Autodesk Fusion 360 part; units mm, degrees
(part 3 of 3)
  line L1894 (31.4632, 18.5996) -> (31.4764, 18.5928)
  line L1895 (31.4764, 18.5928) -> (31.4891, 18.5858)
  line L1896 (31.4891, 18.5858) -> (31.5018, 18.5786)
  line L1897 (31.5018, 18.5786) -> (31.5145, 18.5712)
  line L1898 (31.5145, 18.5712) -> (31.527, 18.5635)
  line L1899 (31.527, 18.5635) -> (31.5394, 18.5556)
  line L1900 (31.5394, 18.5556) -> (31.5516, 18.5475)
  line L1901 (31.5516, 18.5475) -> (31.5637, 18.5392)
  line L1902 (31.5637, 18.5392) -> (31.5756, 18.5307)
  line L1903 (31.5756, 18.5307) -> (31.5875, 18.522)
  line L1904 (31.5875, 18.522) -> (31.5992, 18.5131)
  line L1905 (31.5992, 18.5131) -> (31.6106, 18.504)
  line L1906 (31.6106, 18.504) -> (31.6219, 18.4946)
  line L1907 (31.6219, 18.4946) -> (31.6331, 18.4851)
  line L1908 (31.6331, 18.4851) -> (31.6439, 18.4754)
  line L1909 (31.6439, 18.4754) -> (31.6547, 18.4655)
  line L1910 (31.6547, 18.4655) -> (31.6656, 18.4554)
  line L1911 (31.6656, 18.4554) -> (31.6759, 18.4451)
  line L1912 (31.6759, 18.4451) -> (31.6862, 18.4347)
  line L1913 (31.6862, 18.4347) -> (31.6963, 18.424)
  line L1914 (31.6963, 18.424) -> (31.7061, 18.4132)
  line L1915 (31.7061, 18.4132) -> (31.7159, 18.4022)
  line L1916 (31.7159, 18.4022) -> (31.7254, 18.3911)
  line L1917 (31.7254, 18.3911) -> (31.7347, 18.3798)
  line L1918 (31.7347, 18.3798) -> (31.7439, 18.3683)
  line L1919 (31.7439, 18.3683) -> (31.7529, 18.3567)
  line L1920 (31.7529, 18.3567) -> (31.7616, 18.3449)
  line L1921 (31.7616, 18.3449) -> (31.7701, 18.3329)
  line L1922 (31.7701, 18.3329) -> (31.7783, 18.3209)
  line L1923 (31.7783, 18.3209) -> (31.7865, 18.3086)
  line L1924 (31.7865, 18.3086) -> (31.7944, 18.2963)
  line L1925 (31.7944, 18.2963) -> (31.8021, 18.2838)
  line L1926 (31.8021, 18.2838) -> (31.8095, 18.2711)
  line L1927 (31.8095, 18.2711) -> (31.8167, 18.2584)
  line L1928 (31.8167, 18.2584) -> (31.8236, 18.2455)
  line L1929 (31.8236, 18.2455) -> (31.8304, 18.2325)
  line L1930 (31.8304, 18.2325) -> (31.837, 18.2194)
  line L1931 (31.837, 18.2194) -> (31.8434, 18.2061)
  line L1932 (31.8434, 18.2061) -> (31.8495, 18.1928)
  line L1933 (31.8495, 18.1928) -> (31.8553, 18.1793)
  line L1934 (31.8553, 18.1793) -> (31.8609, 18.1658)
  line L1935 (31.8609, 18.1658) -> (31.8662, 18.1522)
  line L1936 (31.8662, 18.1522) -> (31.8714, 18.1384)
  line L1937 (31.8714, 18.1384) -> (31.8762, 18.1246)
  line L1938 (31.8762, 18.1246) -> (31.881, 18.1107)
  line L1939 (31.881, 18.1107) -> (31.8852, 18.0967)
  line L1940 (31.8852, 18.0967) -> (31.8894, 18.0827)
  line L1941 (31.8894, 18.0827) -> (31.8934, 18.0685)
  line L1942 (31.8934, 18.0685) -> (31.8971, 18.0543)
  line L1943 (31.8971, 18.0543) -> (31.9005, 18.0401)
  line L1944 (31.9005, 18.0401) -> (31.9037, 18.0258)
  line L1945 (31.9037, 18.0258) -> (31.9066, 18.0114)
  line L1946 (31.9066, 18.0114) -> (31.9093, 17.997)
  line L1947 (31.9093, 17.997) -> (31.9117, 17.9825)
  line L1948 (31.9117, 17.9825) -> (31.9138, 17.968)
  line L1949 (31.9138, 17.968) -> (31.9156, 17.9535)
  line L1950 (31.9156, 17.9535) -> (31.9175, 17.9389)
  line L1951 (31.9175, 17.9389) -> (31.9188, 17.9243)
  line L1952 (31.9188, 17.9243) -> (31.9199, 17.9097)
  line L1953 (31.9199, 17.9097) -> (31.9209, 17.8951)
  line L1954 (31.9209, 17.8951) -> (31.9215, 17.8804)
  line L1955 (31.9215, 17.8804) -> (31.922, 17.8658)
  line L1956 (31.922, 17.8658) -> (31.922, 17.8511)
  line L1957 (31.922, 17.8511) -> (31.922, 6.9304)
  line L1958 (31.922, 6.9304) -> (31.922, 6.9158)
  line L1959 (31.922, 6.9158) -> (31.9215, 6.9011)
  line L1960 (31.9215, 6.9011) -> (31.9209, 6.8865)
  line L1961 (31.9209, 6.8865) -> (31.9199, 6.8718)
  line L1962 (31.9199, 6.8718) -> (31.9188, 6.8572)
  line L1963 (31.9188, 6.8572) -> (31.9175, 6.8426)
  line L1964 (31.9175, 6.8426) -> (31.9156, 6.828)
  line L1965 (31.9156, 6.828) -> (31.9138, 6.8135)
  line L1966 (31.9138, 6.8135) -> (31.9117, 6.799)
  line L1967 (31.9117, 6.799) -> (31.9093, 6.7846)
  line L1968 (31.9093, 6.7846) -> (31.9066, 6.7701)
  line L1969 (31.9066, 6.7701) -> (31.9037, 6.7558)
  line L1970 (31.9037, 6.7558) -> (31.9005, 6.7415)
  line L1971 (31.9005, 6.7415) -> (31.8971, 6.7272)
  line L1972 (31.8971, 6.7272) -> (31.8934, 6.713)
  line L1973 (31.8934, 6.713) -> (31.8894, 6.6989)
  line L1974 (31.8894, 6.6989) -> (31.8852, 6.6848)
  line L1975 (31.8852, 6.6848) -> (31.881, 6.6708)
  line L1976 (31.881, 6.6708) -> (31.8762, 6.6569)
  line L1977 (31.8762, 6.6569) -> (31.8714, 6.6431)
  line L1978 (31.8714, 6.6431) -> (31.8662, 6.6294)
  line L1979 (31.8662, 6.6294) -> (31.8609, 6.6157)
  line L1980 (31.8609, 6.6157) -> (31.8553, 6.6022)
  line L1981 (31.8553, 6.6022) -> (31.8495, 6.5888)
  line L1982 (31.8495, 6.5888) -> (31.8434, 6.5754)
  line L1983 (31.8434, 6.5754) -> (31.837, 6.5622)
  line L1984 (31.837, 6.5622) -> (31.8304, 6.549)
  line L1985 (31.8304, 6.549) -> (31.8236, 6.5361)
  line L1986 (31.8236, 6.5361) -> (31.8167, 6.5232)
  line L1987 (31.8167, 6.5232) -> (31.8095, 6.5104)
  line L1988 (31.8095, 6.5104) -> (31.8021, 6.4978)
  line L1989 (31.8021, 6.4978) -> (31.7944, 6.4853)
  line L1990 (31.7944, 6.4853) -> (31.7865, 6.4729)
  line L1991 (31.7865, 6.4729) -> (31.7783, 6.4607)
  line L1992 (31.7783, 6.4607) -> (31.7701, 6.4486)
  line L1993 (31.7701, 6.4486) -> (31.7616, 6.4367)
  line L1994 (31.7616, 6.4367) -> (31.7529, 6.4249)
  line L1995 (31.7529, 6.4249) -> (31.7439, 6.4132)
  line L1996 (31.7439, 6.4132) -> (31.7347, 6.4018)
  line L1997 (31.7347, 6.4018) -> (31.7254, 6.3905)
  line L1998 (31.7254, 6.3905) -> (31.7159, 6.3793)
  line L1999 (31.7159, 6.3793) -> (31.7061, 6.3683)
  line L2000 (31.7061, 6.3683) -> (31.6963, 6.3575)
  line L2001 (31.6963, 6.3575) -> (31.6862, 6.3469)
  line L2002 (31.6862, 6.3469) -> (31.6759, 6.3364)
  line L2003 (31.6759, 6.3364) -> (31.6656, 6.3261)
  line L2004 (31.6656, 6.3261) -> (31.6547, 6.3161)
  line L2005 (31.6547, 6.3161) -> (31.6439, 6.3062)
  line L2006 (31.6439, 6.3062) -> (31.6331, 6.2964)
  line L2007 (31.6331, 6.2964) -> (31.6219, 6.2869)
  line L2008 (31.6219, 6.2869) -> (31.6106, 6.2776)
  line L2009 (31.6106, 6.2776) -> (31.5992, 6.2685)
  line L2010 (31.5992, 6.2685) -> (31.5875, 6.2595)
  line L2011 (31.5875, 6.2595) -> (31.5756, 6.2508)
  line L2012 (31.5756, 6.2508) -> (31.5637, 6.2423)
  line L2013 (31.5637, 6.2423) -> (31.5516, 6.234)
  line L2014 (31.5516, 6.234) -> (31.5394, 6.2259)
  line L2015 (31.5394, 6.2259) -> (31.527, 6.218)
  line L2016 (31.527, 6.218) -> (31.5145, 6.2104)
  line L2017 (31.5145, 6.2104) -> (31.5018, 6.2029)
  line L2018 (31.5018, 6.2029) -> (31.4891, 6.1957)
  line L2019 (31.4891, 6.1957) -> (31.4764, 6.1887)
  line L2020 (31.4764, 6.1887) -> (31.4632, 6.1819)
  line L2021 (31.4632, 6.1819) -> (31.4502, 6.1754)
  line L2022 (31.4502, 6.1754) -> (31.437, 6.1691)
  line L2023 (31.437, 6.1691) -> (31.4235, 6.163)
  line L2024 (31.4235, 6.163) -> (31.4103, 6.1571)
  line L2025 (31.4103, 6.1571) -> (31.3965, 6.1515)
  line L2026 (31.3965, 6.1515) -> (31.383, 6.1462)
  line L2027 (31.383, 6.1462) -> (31.3693, 6.141)
  line L2028 (31.3693, 6.141) -> (31.3555, 6.1361)
  line L2029 (31.3555, 6.1361) -> (31.3415, 6.1315)
  line L2030 (31.3415, 6.1315) -> (31.3275, 6.1271)
  line L2031 (31.3275, 6.1271) -> (31.3134, 6.1229)
  line L2032 (31.3134, 6.1229) -> (31.2994, 6.119)
  line L2033 (31.2994, 6.119) -> (31.2851, 6.1153)
  line L2034 (31.2851, 6.1153) -> (31.2708, 6.1119)
  line L2035 (31.2708, 6.1119) -> (31.2566, 6.1087)
  line L2036 (31.2566, 6.1087) -> (31.2423, 6.1058)
  line L2037 (31.2423, 6.1058) -> (31.2277, 6.1031)
  line L2038 (31.2277, 6.1031) -> (31.2134, 6.1007)
  line L2039 (31.2134, 6.1007) -> (31.1989, 6.0985)
  line L2040 (31.1989, 6.0985) -> (31.1843, 6.0966)
  line L2041 (31.1843, 6.0966) -> (31.1698, 6.095)
  line L2042 (31.1698, 6.095) -> (31.1552, 6.0936)
  line L2043 (31.1552, 6.0936) -> (31.1404, 6.0924)
  line L2044 (31.1404, 6.0924) -> (31.1258, 6.0915)
  line L2045 (31.1258, 6.0915) -> (31.1113, 6.0909)
  line L2046 (31.1113, 6.0909) -> (31.0965, 6.0905)
  line L2047 (31.0965, 6.0905) -> (31.0819, 6.0904)
  line L2048 (31.0819, 6.0904) -> (3.7802, 6.0904)
  line L2049 (-0.0202, -1.1549) -> (-0.0403, -1.1544)
  line L2050 (-0.0403, -1.1544) -> (-0.0604, -1.1535)
  line L2051 (-0.0604, -1.1535) -> (-0.0806, -1.1523)
  line L2052 (-0.0806, -1.1523) -> (-0.1007, -1.1507)
  line L2053 (-0.1007, -1.1507) -> (-0.1207, -1.1487)
  line L2054 (-0.1207, -1.1487) -> (-0.1408, -1.1465)
  line L2055 (-0.1408, -1.1465) -> (-0.1608, -1.1438)
  line L2056 (-0.1608, -1.1438) -> (-0.1807, -1.1408)
  line L2057 (-0.1807, -1.1408) -> (-0.2006, -1.1375)
  line L2058 (-0.2006, -1.1375) -> (-0.2204, -1.1339)
  line L2059 (-0.2204, -1.1339) -> (-0.2402, -1.1298)
  line L2060 (-0.2402, -1.1298) -> (-0.2598, -1.1255)
  line L2061 (-0.2598, -1.1255) -> (-0.2794, -1.1208)
  line L2062 (-0.2794, -1.1208) -> (-0.299, -1.1157)
  line L2063 (-0.299, -1.1157) -> (-0.3184, -1.1103)
  line L2064 (-0.3184, -1.1103) -> (-0.3377, -1.1046)
  line L2065 (-0.3377, -1.1046) -> (-0.3569, -1.0985)
  line L2066 (-0.3569, -1.0985) -> (-0.3761, -1.0921)
  line L2067 (-0.3761, -1.0921) -> (-0.3951, -1.0854)
  line L2068 (-0.3951, -1.0854) -> (-0.4139, -1.0783)
  line L2069 (-0.4139, -1.0783) -> (-0.4327, -1.071)
  line L2070 (-0.4327, -1.071) -> (-0.4513, -1.0632)
  line L2071 (-0.4513, -1.0632) -> (-0.4698, -1.0552)
  line L2072 (-0.4698, -1.0552) -> (-0.4882, -1.0468)
  line L2073 (-0.4882, -1.0468) -> (-0.5063, -1.0382)
  line L2074 (-0.5063, -1.0382) -> (-0.5244, -1.0292)
  line L2075 (-0.5244, -1.0292) -> (-0.5423, -1.0199)
  line L2076 (-0.5423, -1.0199) -> (-0.56, -1.0102)
  line L2077 (-0.56, -1.0102) -> (-0.5775, -1.0003)
  line L2078 (-0.5775, -1.0003) -> (-0.5949, -0.9901)
  line L2079 (-0.5949, -0.9901) -> (-0.6121, -0.9796)
  line L2080 (-0.6121, -0.9796) -> (-0.6291, -0.9687)
  line L2081 (-0.6291, -0.9687) -> (-0.6459, -0.9576)
  line L2082 (-0.6459, -0.9576) -> (-0.6625, -0.9462)
  line L2083 (-0.6625, -0.9462) -> (-0.6789, -0.9345)
  line L2084 (-0.6789, -0.9345) -> (-0.6951, -0.9225)
  line L2085 (-0.6951, -0.9225) -> (-0.7111, -0.9102)
  line L2086 (-0.7111, -0.9102) -> (-0.7269, -0.8977)
  line L2087 (-0.7269, -0.8977) -> (-0.7425, -0.8848)
  line L2088 (-0.7425, -0.8848) -> (-0.7578, -0.8717)
  line L2089 (-0.7578, -0.8717) -> (-0.7729, -0.8584)
  line L2090 (-0.7729, -0.8584) -> (-0.7878, -0.8448)
  line L2091 (-0.7878, -0.8448) -> (-0.8024, -0.8309)
  line L2092 (-0.8024, -0.8309) -> (-0.8168, -0.8168)
  line L2093 (-0.8168, -0.8168) -> (-0.8309, -0.8024)
  line L2094 (-0.8309, -0.8024) -> (-0.8448, -0.7878)
  line L2095 (-0.8448, -0.7878) -> (-0.8584, -0.7729)
  line L2096 (-0.8584, -0.7729) -> (-0.8717, -0.7578)
  line L2097 (-0.8717, -0.7578) -> (-0.8848, -0.7425)
  line L2098 (-0.8848, -0.7425) -> (-0.8977, -0.7269)
  line L2099 (-0.8977, -0.7269) -> (-0.9102, -0.7111)
  line L2100 (-0.9102, -0.7111) -> (-0.9225, -0.6951)
  line L2101 (-0.9225, -0.6951) -> (-0.9345, -0.6789)
  line L2102 (-0.9345, -0.6789) -> (-0.9462, -0.6625)
  line L2103 (-0.9462, -0.6625) -> (-0.9576, -0.6459)
  line L2104 (-0.9576, -0.6459) -> (-0.9687, -0.6291)
  line L2105 (-0.9687, -0.6291) -> (-0.9796, -0.6121)
  line L2106 (-0.9796, -0.6121) -> (-0.9901, -0.5949)
  line L2107 (-0.9901, -0.5949) -> (-1.0003, -0.5775)
  line L2108 (-1.0003, -0.5775) -> (-1.0102, -0.56)
  line L2109 (-1.0102, -0.56) -> (-1.0199, -0.5423)
  line L2110 (-1.0199, -0.5423) -> (-1.0292, -0.5244)
  line L2111 (-1.0292, -0.5244) -> (-1.0382, -0.5063)
  line L2112 (-1.0382, -0.5063) -> (-1.0468, -0.4882)
  line L2113 (-1.0468, -0.4882) -> (-1.0552, -0.4698)
  line L2114 (-1.0552, -0.4698) -> (-1.0632, -0.4513)
  line L2115 (-1.0632, -0.4513) -> (-1.071, -0.4327)
  line L2116 (-1.071, -0.4327) -> (-1.0783, -0.4139)
  line L2117 (-1.0783, -0.4139) -> (-1.0854, -0.3951)
  line L2118 (-1.0854, -0.3951) -> (-1.0921, -0.3761)
  line L2119 (-1.0921, -0.3761) -> (-1.0985, -0.3569)
  line L2120 (-1.0985, -0.3569) -> (-1.1046, -0.3377)
  line L2121 (-1.1046, -0.3377) -> (-1.1103, -0.3184)
  line L2122 (-1.1103, -0.3184) -> (-1.1157, -0.299)
  line L2123 (-1.1157, -0.299) -> (-1.1208, -0.2794)
  line L2124 (-1.1208, -0.2794) -> (-1.1255, -0.2598)
  line L2125 (-1.1255, -0.2598) -> (-1.1298, -0.2402)
  line L2126 (-1.1298, -0.2402) -> (-1.1339, -0.2204)
  line L2127 (-1.1339, -0.2204) -> (-1.1375, -0.2006)
  line L2128 (-1.1375, -0.2006) -> (-1.1408, -0.1807)
  line L2129 (-1.1408, -0.1807) -> (-1.1438, -0.1608)
  line L2130 (-1.1438, -0.1608) -> (-1.1465, -0.1408)
  line L2131 (-1.1465, -0.1408) -> (-1.1487, -0.1207)
  line L2132 (-1.1487, -0.1207) -> (-1.1507, -0.1007)
  line L2133 (-1.1507, -0.1007) -> (-1.1523, -0.0806)
  line L2134 (-1.1523, -0.0806) -> (-1.1535, -0.0604)
  line L2135 (-1.1535, -0.0604) -> (-1.1544, -0.0403)
  line L2136 (-1.1544, -0.0403) -> (-1.1549, -0.0202)
  line L2137 (-1.1549, -0.0202) -> (-1.1551, 0)
  line L2138 (-1.1551, 0) -> (-1.1549, 0.0202)
  line L2139 (-1.1549, 0.0202) -> (-1.1544, 0.0403)
  line L2140 (-1.1544, 0.0403) -> (-1.1535, 0.0604)
  line L2141 (-1.1535, 0.0604) -> (-1.1523, 0.0806)
  line L2142 (-1.1523, 0.0806) -> (-1.1507, 0.1007)
  line L2143 (-1.1507, 0.1007) -> (-1.1487, 0.1207)
  line L2144 (-1.1487, 0.1207) -> (-1.1465, 0.1408)
  line L2145 (-1.1465, 0.1408) -> (-1.1438, 0.1608)
  line L2146 (-1.1438, 0.1608) -> (-1.1408, 0.1807)
  line L2147 (-1.1408, 0.1807) -> (-1.1375, 0.2006)
  line L2148 (-1.1375, 0.2006) -> (-1.1339, 0.2204)
  line L2149 (-1.1339, 0.2204) -> (-1.1298, 0.2402)
  line L2150 (-1.1298, 0.2402) -> (-1.1255, 0.2598)
  line L2151 (-1.1255, 0.2598) -> (-1.1208, 0.2794)
  line L2152 (-1.1208, 0.2794) -> (-1.1157, 0.299)
  line L2153 (-1.1157, 0.299) -> (-1.1103, 0.3184)
  line L2154 (-1.1103, 0.3184) -> (-1.1046, 0.3377)
  line L2155 (-1.1046, 0.3377) -> (-1.0985, 0.3569)
  line L2156 (-1.0985, 0.3569) -> (-1.0921, 0.3761)
  line L2157 (-1.0921, 0.3761) -> (-1.0854, 0.3951)
  line L2158 (-1.0854, 0.3951) -> (-1.0783, 0.4139)
  line L2159 (-1.0783, 0.4139) -> (-1.071, 0.4327)
  line L2160 (-1.071, 0.4327) -> (-1.0632, 0.4513)
  line L2161 (-1.0632, 0.4513) -> (-1.0552, 0.4698)
  line L2162 (-1.0552, 0.4698) -> (-1.0468, 0.4882)
  line L2163 (-1.0468, 0.4882) -> (-1.0382, 0.5063)
  line L2164 (-1.0382, 0.5063) -> (-1.0292, 0.5244)
  line L2165 (-1.0292, 0.5244) -> (-1.0199, 0.5423)
  line L2166 (-1.0199, 0.5423) -> (-1.0102, 0.56)
  line L2167 (-1.0102, 0.56) -> (-1.0003, 0.5775)
  line L2168 (-1.0003, 0.5775) -> (-0.9901, 0.5949)
  line L2169 (-0.9901, 0.5949) -> (-0.9796, 0.6121)
  line L2170 (-0.9796, 0.6121) -> (-0.9687, 0.6291)
  line L2171 (-0.9687, 0.6291) -> (-0.9576, 0.6459)
  line L2172 (-0.9576, 0.6459) -> (-0.9462, 0.6625)
  line L2173 (-0.9462, 0.6625) -> (-0.9345, 0.6789)
  line L2174 (-0.9345, 0.6789) -> (-0.9225, 0.6951)
  line L2175 (-0.9225, 0.6951) -> (-0.9102, 0.7111)
  line L2176 (-0.9102, 0.7111) -> (-0.8977, 0.7269)
  line L2177 (-0.8977, 0.7269) -> (-0.8848, 0.7425)
  line L2178 (-0.8848, 0.7425) -> (-0.8717, 0.7578)
  line L2179 (-0.8717, 0.7578) -> (-0.8584, 0.7729)
  line L2180 (-0.8584, 0.7729) -> (-0.8448, 0.7878)
  line L2181 (-0.8448, 0.7878) -> (-0.8309, 0.8024)
  line L2182 (-0.8309, 0.8024) -> (-0.8168, 0.8168)
  line L2183 (-0.8168, 0.8168) -> (-0.8024, 0.8309)
  line L2184 (-0.8024, 0.8309) -> (-0.7878, 0.8448)
  line L2185 (-0.7878, 0.8448) -> (-0.7729, 0.8584)
  line L2186 (-0.7729, 0.8584) -> (-0.7578, 0.8717)
  line L2187 (-0.7578, 0.8717) -> (-0.7425, 0.8848)
  line L2188 (-0.7425, 0.8848) -> (-0.7269, 0.8977)
  line L2189 (-0.7269, 0.8977) -> (-0.7111, 0.9102)
  line L2190 (-0.7111, 0.9102) -> (-0.6951, 0.9225)
  line L2191 (-0.6951, 0.9225) -> (-0.6789, 0.9345)
  line L2192 (-0.6789, 0.9345) -> (-0.6625, 0.9462)
  line L2193 (-0.6625, 0.9462) -> (-0.6459, 0.9576)
  line L2194 (-0.6459, 0.9576) -> (-0.6291, 0.9687)
  line L2195 (-0.6291, 0.9687) -> (-0.6121, 0.9796)
  line L2196 (-0.6121, 0.9796) -> (-0.5949, 0.9901)
  line L2197 (-0.5949, 0.9901) -> (-0.5775, 1.0003)
  line L2198 (-0.5775, 1.0003) -> (-0.56, 1.0102)
  line L2199 (-0.56, 1.0102) -> (-0.5423, 1.0199)
  line L2200 (-0.5423, 1.0199) -> (-0.5244, 1.0292)
  line L2201 (-0.5244, 1.0292) -> (-0.5063, 1.0382)
  line L2202 (-0.5063, 1.0382) -> (-0.4882, 1.0468)
  line L2203 (-0.4882, 1.0468) -> (-0.4698, 1.0552)
  line L2204 (-0.4698, 1.0552) -> (-0.4513, 1.0632)
  line L2205 (-0.4513, 1.0632) -> (-0.4327, 1.071)
  line L2206 (-0.4327, 1.071) -> (-0.4139, 1.0783)
  line L2207 (-0.4139, 1.0783) -> (-0.3951, 1.0854)
  line L2208 (-0.3951, 1.0854) -> (-0.3761, 1.0921)
  line L2209 (-0.3761, 1.0921) -> (-0.3569, 1.0985)
  line L2210 (-0.3569, 1.0985) -> (-0.3377, 1.1046)
  line L2211 (-0.3377, 1.1046) -> (-0.3184, 1.1103)
  line L2212 (-0.3184, 1.1103) -> (-0.299, 1.1157)
  line L2213 (-0.299, 1.1157) -> (-0.2794, 1.1208)
  line L2214 (-0.2794, 1.1208) -> (-0.2598, 1.1255)
  line L2215 (-0.2598, 1.1255) -> (-0.2402, 1.1298)
  line L2216 (-0.2402, 1.1298) -> (-0.2204, 1.1339)
  line L2217 (-0.2204, 1.1339) -> (-0.2006, 1.1375)
  line L2218 (-0.2006, 1.1375) -> (-0.1807, 1.1408)
  line L2219 (-0.1807, 1.1408) -> (-0.1608, 1.1438)
  line L2220 (-0.1608, 1.1438) -> (-0.1408, 1.1465)
  line L2221 (-0.1408, 1.1465) -> (-0.1207, 1.1487)
  line L2222 (-0.1207, 1.1487) -> (-0.1007, 1.1507)
  line L2223 (-0.1007, 1.1507) -> (-0.0806, 1.1523)
  line L2224 (-0.0806, 1.1523) -> (-0.0604, 1.1535)
  line L2225 (-0.0604, 1.1535) -> (-0.0403, 1.1544)
  line L2226 (-0.0403, 1.1544) -> (-0.0202, 1.1549)
  line L2227 (-0.0202, 1.1549) -> (0, 1.1551)
  line L2228 (0, 1.1551) -> (0.0202, 1.1549)
  line L2229 (0.0202, 1.1549) -> (0.0403, 1.1544)
  line L2230 (0.0403, 1.1544) -> (0.0604, 1.1535)
  line L2231 (0.0604, 1.1535) -> (0.0806, 1.1523)
  line L2232 (0.0806, 1.1523) -> (0.1007, 1.1507)
  line L2233 (0.1007, 1.1507) -> (0.1207, 1.1487)
  line L2234 (0.1207, 1.1487) -> (0.1408, 1.1465)
  line L2235 (0.1408, 1.1465) -> (0.1608, 1.1438)
  line L2236 (0.1608, 1.1438) -> (0.1807, 1.1408)
  line L2237 (0.1807, 1.1408) -> (0.2006, 1.1375)
  line L2238 (0.2006, 1.1375) -> (0.2204, 1.1339)
  line L2239 (0.2204, 1.1339) -> (0.2402, 1.1298)
  line L2240 (0.2402, 1.1298) -> (0.2598, 1.1255)
  line L2241 (0.2598, 1.1255) -> (0.2794, 1.1208)
  line L2242 (0.2794, 1.1208) -> (0.299, 1.1157)
  line L2243 (0.299, 1.1157) -> (0.3184, 1.1103)
  line L2244 (0.3184, 1.1103) -> (0.3377, 1.1046)
  line L2245 (0.3377, 1.1046) -> (0.3569, 1.0985)
  line L2246 (0.3569, 1.0985) -> (0.3761, 1.0921)
  line L2247 (0.3761, 1.0921) -> (0.3951, 1.0854)
  line L2248 (0.3951, 1.0854) -> (0.4139, 1.0783)
  line L2249 (0.4139, 1.0783) -> (0.4327, 1.071)
  line L2250 (0.4327, 1.071) -> (0.4513, 1.0632)
  line L2251 (0.4513, 1.0632) -> (0.4698, 1.0552)
  line L2252 (0.4698, 1.0552) -> (0.4882, 1.0468)
  line L2253 (0.4882, 1.0468) -> (0.5063, 1.0382)
  line L2254 (0.5063, 1.0382) -> (0.5244, 1.0292)
  line L2255 (0.5244, 1.0292) -> (0.5423, 1.0199)
  line L2256 (0.5423, 1.0199) -> (0.56, 1.0102)
  line L2257 (0.56, 1.0102) -> (0.5775, 1.0003)
  line L2258 (0.5775, 1.0003) -> (0.5949, 0.9901)
  line L2259 (0.5949, 0.9901) -> (0.6121, 0.9796)
  line L2260 (0.6121, 0.9796) -> (0.6291, 0.9687)
  line L2261 (0.6291, 0.9687) -> (0.6459, 0.9576)
  line L2262 (0.6459, 0.9576) -> (0.6625, 0.9462)
  line L2263 (0.6625, 0.9462) -> (0.6789, 0.9345)
  line L2264 (0.6789, 0.9345) -> (0.6951, 0.9225)
  line L2265 (0.6951, 0.9225) -> (0.7111, 0.9102)
  line L2266 (0.7111, 0.9102) -> (0.7269, 0.8977)
  line L2267 (0.7269, 0.8977) -> (0.7425, 0.8848)
  line L2268 (0.7425, 0.8848) -> (0.7578, 0.8717)
  line L2269 (0.7578, 0.8717) -> (0.7729, 0.8584)
  line L2270 (0.7729, 0.8584) -> (0.7878, 0.8448)
  line L2271 (0.7878, 0.8448) -> (0.8024, 0.8309)
  line L2272 (0.8024, 0.8309) -> (0.8168, 0.8168)
  line L2273 (0.8168, 0.8168) -> (0.8309, 0.8024)
  line L2274 (0.8309, 0.8024) -> (0.8448, 0.7878)
  line L2275 (0.8448, 0.7878) -> (0.8584, 0.7729)
  line L2276 (0.8584, 0.7729) -> (0.8717, 0.7578)
  line L2277 (0.8717, 0.7578) -> (0.8848, 0.7425)
  line L2278 (0.8848, 0.7425) -> (0.8977, 0.7269)
  line L2279 (0.8977, 0.7269) -> (0.9102, 0.7111)
  line L2280 (0.9102, 0.7111) -> (0.9225, 0.6951)
  line L2281 (0.9225, 0.6951) -> (0.9345, 0.6789)
  line L2282 (0.9345, 0.6789) -> (0.9462, 0.6625)
  line L2283 (0.9462, 0.6625) -> (0.9576, 0.6459)
  line L2284 (0.9576, 0.6459) -> (0.9687, 0.6291)
  line L2285 (0.9687, 0.6291) -> (0.9796, 0.6121)
  line L2286 (0.9796, 0.6121) -> (0.9901, 0.5949)
  line L2287 (0.9901, 0.5949) -> (1.0003, 0.5775)
  line L2288 (1.0003, 0.5775) -> (1.0102, 0.56)
  line L2289 (1.0102, 0.56) -> (1.0199, 0.5423)
  line L2290 (1.0199, 0.5423) -> (1.0292, 0.5244)
  line L2291 (1.0292, 0.5244) -> (1.0382, 0.5063)
  line L2292 (1.0382, 0.5063) -> (1.0468, 0.4882)
  line L2293 (1.0468, 0.4882) -> (1.0552, 0.4698)
  line L2294 (1.0552, 0.4698) -> (1.0632, 0.4513)
  line L2295 (1.0632, 0.4513) -> (1.071, 0.4327)
  line L2296 (1.071, 0.4327) -> (1.0783, 0.4139)
  line L2297 (1.0783, 0.4139) -> (1.0854, 0.3951)
  line L2298 (1.0854, 0.3951) -> (1.0921, 0.3761)
  line L2299 (1.0921, 0.3761) -> (1.0985, 0.3569)
  line L2300 (1.0985, 0.3569) -> (1.1046, 0.3377)
  line L2301 (1.1046, 0.3377) -> (1.1103, 0.3184)
  line L2302 (1.1103, 0.3184) -> (1.1157, 0.299)
  line L2303 (1.1157, 0.299) -> (1.1208, 0.2794)
  line L2304 (1.1208, 0.2794) -> (1.1255, 0.2598)
  line L2305 (1.1255, 0.2598) -> (1.1298, 0.2402)
  line L2306 (1.1298, 0.2402) -> (1.1339, 0.2204)
  line L2307 (1.1339, 0.2204) -> (1.1375, 0.2006)
  line L2308 (1.1375, 0.2006) -> (1.1408, 0.1807)
  line L2309 (1.1408, 0.1807) -> (1.1438, 0.1608)
  line L2310 (1.1438, 0.1608) -> (1.1465, 0.1408)
  line L2311 (1.1465, 0.1408) -> (1.1487, 0.1207)
  line L2312 (1.1487, 0.1207) -> (1.1507, 0.1007)
  line L2313 (1.1507, 0.1007) -> (1.1523, 0.0806)
  line L2314 (1.1523, 0.0806) -> (1.1535, 0.0604)
  line L2315 (1.1535, 0.0604) -> (1.1544, 0.0403)
  line L2316 (1.1544, 0.0403) -> (1.1549, 0.0202)
  line L2317 (1.1549, 0.0202) -> (1.1551, 0)
  line L2318 (1.1551, 0) -> (1.1549, -0.0202)
  line L2319 (1.1549, -0.0202) -> (1.1544, -0.0403)
  line L2320 (1.1544, -0.0403) -> (1.1535, -0.0604)
  line L2321 (1.1535, -0.0604) -> (1.1523, -0.0806)
  line L2322 (1.1523, -0.0806) -> (1.1507, -0.1007)
  line L2323 (1.1507, -0.1007) -> (1.1487, -0.1207)
  line L2324 (1.1487, -0.1207) -> (1.1465, -0.1408)
  line L2325 (1.1465, -0.1408) -> (1.1438, -0.1608)
  line L2326 (1.1438, -0.1608) -> (1.1408, -0.1807)
  line L2327 (1.1408, -0.1807) -> (1.1375, -0.2006)
  line L2328 (1.1375, -0.2006) -> (1.1339, -0.2204)
  line L2329 (1.1339, -0.2204) -> (1.1298, -0.2402)
  line L2330 (1.1298, -0.2402) -> (1.1255, -0.2598)
  line L2331 (1.1255, -0.2598) -> (1.1208, -0.2794)
  line L2332 (1.1208, -0.2794) -> (1.1157, -0.299)
  line L2333 (1.1157, -0.299) -> (1.1103, -0.3184)
  line L2334 (1.1103, -0.3184) -> (1.1046, -0.3377)
  line L2335 (1.1046, -0.3377) -> (1.0985, -0.3569)
  line L2336 (1.0985, -0.3569) -> (1.0921, -0.3761)
  line L2337 (1.0921, -0.3761) -> (1.0854, -0.3951)
  line L2338 (1.0854, -0.3951) -> (1.0783, -0.4139)
  line L2339 (1.0783, -0.4139) -> (1.071, -0.4327)
  line L2340 (1.071, -0.4327) -> (1.0632, -0.4513)
  line L2341 (1.0632, -0.4513) -> (1.0552, -0.4698)
  line L2342 (1.0552, -0.4698) -> (1.0468, -0.4882)
  line L2343 (1.0468, -0.4882) -> (1.0382, -0.5063)
  line L2344 (1.0382, -0.5063) -> (1.0292, -0.5244)
  line L2345 (1.0292, -0.5244) -> (1.0199, -0.5423)
  line L2346 (1.0199, -0.5423) -> (1.0102, -0.56)
  line L2347 (1.0102, -0.56) -> (1.0003, -0.5775)
  line L2348 (1.0003, -0.5775) -> (0.9901, -0.5949)
  line L2349 (0.9901, -0.5949) -> (0.9796, -0.6121)
  line L2350 (0.9796, -0.6121) -> (0.9687, -0.6291)
  line L2351 (0.9687, -0.6291) -> (0.9576, -0.6459)
  line L2352 (0.9576, -0.6459) -> (0.9462, -0.6625)
  line L2353 (0.9462, -0.6625) -> (0.9345, -0.6789)
  line L2354 (0.9345, -0.6789) -> (0.9225, -0.6951)
  line L2355 (0.9225, -0.6951) -> (0.9102, -0.7111)
  line L2356 (0.9102, -0.7111) -> (0.8977, -0.7269)
  line L2357 (0.8977, -0.7269) -> (0.8848, -0.7425)
  line L2358 (0.8848, -0.7425) -> (0.8717, -0.7578)
  line L2359 (0.8717, -0.7578) -> (0.8584, -0.7729)
  line L2360 (0.8584, -0.7729) -> (0.8448, -0.7878)
  line L2361 (0.8448, -0.7878) -> (0.8309, -0.8024)
  line L2362 (0.8309, -0.8024) -> (0.8168, -0.8168)
  line L2363 (0.8168, -0.8168) -> (0.8024, -0.8309)
  line L2364 (0.8024, -0.8309) -> (0.7878, -0.8448)
  line L2365 (0.7878, -0.8448) -> (0.7729, -0.8584)
  line L2366 (0.7729, -0.8584) -> (0.7578, -0.8717)
  line L2367 (0.7578, -0.8717) -> (0.7425, -0.8848)
  line L2368 (0.7425, -0.8848) -> (0.7269, -0.8977)
  line L2369 (0.7269, -0.8977) -> (0.7111, -0.9102)
  line L2370 (0.7111, -0.9102) -> (0.6951, -0.9225)
  line L2371 (0.6951, -0.9225) -> (0.6789, -0.9345)
  line L2372 (0.6789, -0.9345) -> (0.6625, -0.9462)
  line L2373 (0.6625, -0.9462) -> (0.6459, -0.9576)
  line L2374 (0.6459, -0.9576) -> (0.6291, -0.9687)
  line L2375 (0.6291, -0.9687) -> (0.6121, -0.9796)
  line L2376 (0.6121, -0.9796) -> (0.5949, -0.9901)
  line L2377 (0.5949, -0.9901) -> (0.5775, -1.0003)
  line L2378 (0.5775, -1.0003) -> (0.56, -1.0102)
  line L2379 (0.56, -1.0102) -> (0.5423, -1.0199)
  line L2380 (0.5423, -1.0199) -> (0.5244, -1.0292)
  line L2381 (0.5244, -1.0292) -> (0.5063, -1.0382)
  line L2382 (0.5063, -1.0382) -> (0.4882, -1.0468)
  line L2383 (0.4882, -1.0468) -> (0.4698, -1.0552)
  line L2384 (0.4698, -1.0552) -> (0.4513, -1.0632)
  line L2385 (0.4513, -1.0632) -> (0.4327, -1.071)
  line L2386 (0.4327, -1.071) -> (0.4139, -1.0783)
  line L2387 (0.4139, -1.0783) -> (0.3951, -1.0854)
  line L2388 (0.3951, -1.0854) -> (0.3761, -1.0921)
  line L2389 (0.3761, -1.0921) -> (0.3569, -1.0985)
  line L2390 (0.3569, -1.0985) -> (0.3377, -1.1046)
  line L2391 (0.3377, -1.1046) -> (0.3184, -1.1103)
  line L2392 (0.3184, -1.1103) -> (0.299, -1.1157)
  line L2393 (0.299, -1.1157) -> (0.2794, -1.1208)
  line L2394 (0.2794, -1.1208) -> (0.2598, -1.1255)
  line L2395 (0.2598, -1.1255) -> (0.2402, -1.1298)
  line L2396 (0.2402, -1.1298) -> (0.2204, -1.1339)
  line L2397 (0.2204, -1.1339) -> (0.2006, -1.1375)
  line L2398 (0.2006, -1.1375) -> (0.1807, -1.1408)
  line L2399 (0.1807, -1.1408) -> (0.1608, -1.1438)
  line L2400 (0.1608, -1.1438) -> (0.1408, -1.1465)
  line L2401 (0.1408, -1.1465) -> (0.1207, -1.1487)
  line L2402 (0.1207, -1.1487) -> (0.1007, -1.1507)
  line L2403 (0.1007, -1.1507) -> (0.0806, -1.1523)
  line L2404 (0.0806, -1.1523) -> (0.0604, -1.1535)
  line L2405 (0.0604, -1.1535) -> (0.0403, -1.1544)
  line L2406 (0.0403, -1.1544) -> (0.0202, -1.1549)
  line L2407 (0.0202, -1.1549) -> (0, -1.1551)
  line L2408 (0, -1.1551) -> (-0.0202, -1.1549)
  line L2409 (34.6321, -1.1549) -> (34.6117, -1.1544)
  line L2410 (34.6117, -1.1544) -> (34.5916, -1.1535)
  line L2411 (34.5916, -1.1535) -> (34.5715, -1.1523)
  line L2412 (34.5715, -1.1523) -> (34.5514, -1.1507)
  line L2413 (34.5514, -1.1507) -> (34.5313, -1.1487)
  line L2414 (34.5313, -1.1487) -> (34.5115, -1.1465)
  line L2415 (34.5115, -1.1465) -> (34.4913, -1.1438)
  line L2416 (34.4913, -1.1438) -> (34.4715, -1.1408)
  line L2417 (34.4715, -1.1408) -> (34.4517, -1.1375)
  line L2418 (34.4517, -1.1375) -> (34.4318, -1.1339)
  line L2419 (34.4318, -1.1339) -> (34.412, -1.1298)
  line L2420 (34.412, -1.1298) -> (34.3924, -1.1255)
  line L2421 (34.3924, -1.1255) -> (34.3728, -1.1208)
  line L2422 (34.3728, -1.1208) -> (34.3532, -1.1157)
  line L2423 (34.3532, -1.1157) -> (34.3337, -1.1103)
  line L2424 (34.3337, -1.1103) -> (34.3143, -1.1046)
  line L2425 (34.3143, -1.1046) -> (34.2953, -1.0985)
  line L2426 (34.2953, -1.0985) -> (34.276, -1.0921)
  line L2427 (34.276, -1.0921) -> (34.2572, -1.0854)
  line L2428 (34.2572, -1.0854) -> (34.2381, -1.0783)
  line L2429 (34.2381, -1.0783) -> (34.2194, -1.071)
  line L2430 (34.2194, -1.071) -> (34.2008, -1.0632)
  line L2431 (34.2008, -1.0632) -> (34.1823, -1.0552)
  line L2432 (34.1823, -1.0552) -> (34.1641, -1.0468)
  line L2433 (34.1641, -1.0468) -> (34.1458, -1.0382)
  line L2434 (34.1458, -1.0382) -> (34.1278, -1.0292)
  line L2435 (34.1278, -1.0292) -> (34.1098, -1.0199)
  line L2436 (34.1098, -1.0199) -> (34.0921, -1.0102)
  line L2437 (34.0921, -1.0102) -> (34.0746, -1.0003)
  line L2438 (34.0746, -1.0003) -> (34.0572, -0.9901)
  line L2439 (34.0572, -0.9901) -> (34.04, -0.9796)
  line L2440 (34.04, -0.9796) -> (34.023, -0.9687)
  line L2441 (34.023, -0.9687) -> (34.0064, -0.9576)
  line L2442 (34.0064, -0.9576) -> (33.9897, -0.9462)
  line L2443 (33.9897, -0.9462) -> (33.9733, -0.9345)
  line L2444 (33.9733, -0.9345) -> (33.9569, -0.9225)
  line L2445 (33.9569, -0.9225) -> (33.941, -0.9102)
  line L2446 (33.941, -0.9102) -> (33.9251, -0.8977)
  line L2447 (33.9251, -0.8977) -> (33.9098, -0.8848)
  line L2448 (33.9098, -0.8848) -> (33.8944, -0.8717)
  line L2449 (33.8944, -0.8717) -> (33.8794, -0.8584)
  line L2450 (33.8794, -0.8584) -> (33.8643, -0.8448)
  line L2451 (33.8643, -0.8448) -> (33.8497, -0.8309)
  line L2452 (33.8497, -0.8309) -> (33.8354, -0.8168)
  line L2453 (33.8354, -0.8168) -> (33.8212, -0.8024)
  line L2454 (33.8212, -0.8024) -> (33.8074, -0.7878)
  line L2455 (33.8074, -0.7878) -> (33.7936, -0.7729)
  line L2456 (33.7936, -0.7729) -> (33.7804, -0.7578)
  line L2457 (33.7804, -0.7578) -> (33.7672, -0.7425)
  line L2458 (33.7672, -0.7425) -> (33.7545, -0.7269)
  line L2459 (33.7545, -0.7269) -> (33.742, -0.7111)
  line L2460 (33.742, -0.7111) -> (33.7296, -0.6951)
  line L2461 (33.7296, -0.6951) -> (33.7177, -0.6789)
  line L2462 (33.7177, -0.6789) -> (33.7061, -0.6625)
  line L2463 (33.7061, -0.6625) -> (33.6944, -0.6459)
  line L2464 (33.6944, -0.6459) -> (33.6833, -0.6291)
  line L2465 (33.6833, -0.6291) -> (33.6725, -0.6121)
  line L2466 (33.6725, -0.6121) -> (33.6621, -0.5949)
  line L2467 (33.6621, -0.5949) -> (33.6518, -0.5775)
  line L2468 (33.6518, -0.5775) -> (33.6418, -0.56)
  line L2469 (33.6418, -0.56) -> (33.6322, -0.5423)
  line L2470 (33.6322, -0.5423) -> (33.623, -0.5244)
  line L2471 (33.623, -0.5244) -> (33.614, -0.5063)
  line L2472 (33.614, -0.5063) -> (33.6053, -0.4882)
  line L2473 (33.6053, -0.4882) -> (33.5971, -0.4698)
  line L2474 (33.5971, -0.4698) -> (33.5889, -0.4513)
  line L2475 (33.5889, -0.4513) -> (33.5812, -0.4327)
  line L2476 (33.5812, -0.4327) -> (33.5738, -0.4139)
  line L2477 (33.5738, -0.4139) -> (33.5666, -0.3951)
  line L2478 (33.5666, -0.3951) -> (33.56, -0.3761)
  line L2479 (33.56, -0.3761) -> (33.5537, -0.3569)
  line L2480 (33.5537, -0.3569) -> (33.5476, -0.3377)
  line L2481 (33.5476, -0.3377) -> (33.5418, -0.3184)
  line L2482 (33.5418, -0.3184) -> (33.5365, -0.299)
  line L2483 (33.5365, -0.299) -> (33.5314, -0.2794)
  line L2484 (33.5314, -0.2794) -> (33.5267, -0.2598)
  line L2485 (33.5267, -0.2598) -> (33.5224, -0.2402)
  line L2486 (33.5224, -0.2402) -> (33.5182, -0.2204)
  line L2487 (33.5182, -0.2204) -> (33.5145, -0.2006)
  line L2488 (33.5145, -0.2006) -> (33.5113, -0.1807)
  line L2489 (33.5113, -0.1807) -> (33.5084, -0.1608)
  line L2490 (33.5084, -0.1608) -> (33.5058, -0.1408)
  line L2491 (33.5058, -0.1408) -> (33.5034, -0.1207)
  line L2492 (33.5034, -0.1207) -> (33.5015, -0.1007)
  line L2493 (33.5015, -0.1007) -> (33.5, -0.0806)
  line L2494 (33.5, -0.0806) -> (33.4986, -0.0604)
  line L2495 (33.4986, -0.0604) -> (33.4978, -0.0403)
  line L2496 (33.4978, -0.0403) -> (33.4973, -0.0202)
  line L2497 (33.4973, -0.0202) -> (33.497, 0)
  line L2498 (33.497, 0) -> (33.4973, 0.0202)
  line L2499 (33.4973, 0.0202) -> (33.4978, 0.0403)
  line L2500 (33.4978, 0.0403) -> (33.4986, 0.0604)
  line L2501 (33.4986, 0.0604) -> (33.5, 0.0806)
  line L2502 (33.5, 0.0806) -> (33.5015, 0.1007)
  line L2503 (33.5015, 0.1007) -> (33.5034, 0.1207)
  line L2504 (33.5034, 0.1207) -> (33.5058, 0.1408)
  line L2505 (33.5058, 0.1408) -> (33.5084, 0.1608)
  line L2506 (33.5084, 0.1608) -> (33.5113, 0.1807)
  line L2507 (33.5113, 0.1807) -> (33.5145, 0.2006)
  line L2508 (33.5145, 0.2006) -> (33.5182, 0.2204)
  line L2509 (33.5182, 0.2204) -> (33.5224, 0.2402)
  line L2510 (33.5224, 0.2402) -> (33.5267, 0.2598)
  line L2511 (33.5267, 0.2598) -> (33.5314, 0.2794)
  line L2512 (33.5314, 0.2794) -> (33.5365, 0.299)
  line L2513 (33.5365, 0.299) -> (33.5418, 0.3184)
  line L2514 (33.5418, 0.3184) -> (33.5476, 0.3377)
  line L2515 (33.5476, 0.3377) -> (33.5537, 0.3569)
  line L2516 (33.5537, 0.3569) -> (33.56, 0.3761)
  line L2517 (33.56, 0.3761) -> (33.5666, 0.3951)
  line L2518 (33.5666, 0.3951) -> (33.5738, 0.4139)
  line L2519 (33.5738, 0.4139) -> (33.5812, 0.4327)
  line L2520 (33.5812, 0.4327) -> (33.5889, 0.4513)
  line L2521 (33.5889, 0.4513) -> (33.5971, 0.4698)
  line L2522 (33.5971, 0.4698) -> (33.6053, 0.4882)
  line L2523 (33.6053, 0.4882) -> (33.614, 0.5063)
  line L2524 (33.614, 0.5063) -> (33.623, 0.5244)
  line L2525 (33.623, 0.5244) -> (33.6322, 0.5423)
  line L2526 (33.6322, 0.5423) -> (33.6418, 0.56)
  line L2527 (33.6418, 0.56) -> (33.6518, 0.5775)
  line L2528 (33.6518, 0.5775) -> (33.6621, 0.5949)
  line L2529 (33.6621, 0.5949) -> (33.6725, 0.6121)
  line L2530 (33.6725, 0.6121) -> (33.6833, 0.6291)
  line L2531 (33.6833, 0.6291) -> (33.6944, 0.6459)
  line L2532 (33.6944, 0.6459) -> (33.7061, 0.6625)
  line L2533 (33.7061, 0.6625) -> (33.7177, 0.6789)
  line L2534 (33.7177, 0.6789) -> (33.7296, 0.6951)
  line L2535 (33.7296, 0.6951) -> (33.742, 0.7111)
  line L2536 (33.742, 0.7111) -> (33.7545, 0.7269)
  line L2537 (33.7545, 0.7269) -> (33.7672, 0.7425)
  line L2538 (33.7672, 0.7425) -> (33.7804, 0.7578)
  line L2539 (33.7804, 0.7578) -> (33.7936, 0.7729)
  line L2540 (33.7936, 0.7729) -> (33.8074, 0.7878)
  line L2541 (33.8074, 0.7878) -> (33.8212, 0.8024)
  line L2542 (33.8212, 0.8024) -> (33.8354, 0.8168)
  line L2543 (33.8354, 0.8168) -> (33.8497, 0.8309)
  line L2544 (33.8497, 0.8309) -> (33.8643, 0.8448)
  line L2545 (33.8643, 0.8448) -> (33.8794, 0.8584)
  line L2546 (33.8794, 0.8584) -> (33.8944, 0.8717)
  line L2547 (33.8944, 0.8717) -> (33.9098, 0.8848)
  line L2548 (33.9098, 0.8848) -> (33.9251, 0.8977)
  line L2549 (33.9251, 0.8977) -> (33.941, 0.9102)
  line L2550 (33.941, 0.9102) -> (33.9569, 0.9225)
  line L2551 (33.9569, 0.9225) -> (33.9733, 0.9345)
  line L2552 (33.9733, 0.9345) -> (33.9897, 0.9462)
  line L2553 (33.9897, 0.9462) -> (34.0064, 0.9576)
  line L2554 (34.0064, 0.9576) -> (34.023, 0.9687)
  line L2555 (34.023, 0.9687) -> (34.04, 0.9796)
  line L2556 (34.04, 0.9796) -> (34.0572, 0.9901)
  line L2557 (34.0572, 0.9901) -> (34.0746, 1.0003)
  line L2558 (34.0746, 1.0003) -> (34.0921, 1.0102)
  line L2559 (34.0921, 1.0102) -> (34.1098, 1.0199)
  line L2560 (34.1098, 1.0199) -> (34.1278, 1.0292)
  line L2561 (34.1278, 1.0292) -> (34.1458, 1.0382)
  line L2562 (34.1458, 1.0382) -> (34.1641, 1.0468)
  line L2563 (34.1641, 1.0468) -> (34.1823, 1.0552)
  line L2564 (34.1823, 1.0552) -> (34.2008, 1.0632)
  line L2565 (34.2008, 1.0632) -> (34.2194, 1.071)
  line L2566 (34.2194, 1.071) -> (34.2381, 1.0783)
  line L2567 (34.2381, 1.0783) -> (34.2572, 1.0854)
  line L2568 (34.2572, 1.0854) -> (34.276, 1.0921)
  line L2569 (34.276, 1.0921) -> (34.2953, 1.0985)
  line L2570 (34.2953, 1.0985) -> (34.3143, 1.1046)
  line L2571 (34.3143, 1.1046) -> (34.3337, 1.1103)
  line L2572 (34.3337, 1.1103) -> (34.3532, 1.1157)
  line L2573 (34.3532, 1.1157) -> (34.3728, 1.1208)
  line L2574 (34.3728, 1.1208) -> (34.3924, 1.1255)
  line L2575 (34.3924, 1.1255) -> (34.412, 1.1298)
  line L2576 (34.412, 1.1298) -> (34.4318, 1.1339)
  line L2577 (34.4318, 1.1339) -> (34.4517, 1.1375)
  line L2578 (34.4517, 1.1375) -> (34.4715, 1.1408)
  line L2579 (34.4715, 1.1408) -> (34.4913, 1.1438)
  line L2580 (34.4913, 1.1438) -> (34.5115, 1.1465)
  line L2581 (34.5115, 1.1465) -> (34.5313, 1.1487)
  line L2582 (34.5313, 1.1487) -> (34.5514, 1.1507)
  line L2583 (34.5514, 1.1507) -> (34.5715, 1.1523)
  line L2584 (34.5715, 1.1523) -> (34.5916, 1.1535)
  line L2585 (34.5916, 1.1535) -> (34.6117, 1.1544)
  line L2586 (34.6117, 1.1544) -> (34.6321, 1.1549)
  line L2587 (34.6321, 1.1549) -> (34.6522, 1.1551)
  line L2588 (34.6522, 1.1551) -> (34.6723, 1.1549)
  line L2589 (34.6723, 1.1549) -> (34.6924, 1.1544)
  line L2590 (34.6924, 1.1544) -> (34.7125, 1.1535)
  line L2591 (34.7125, 1.1535) -> (34.7326, 1.1523)
  line L2592 (34.7326, 1.1523) -> (34.7528, 1.1507)
  line L2593 (34.7528, 1.1507) -> (34.7729, 1.1487)
  line L2594 (34.7729, 1.1487) -> (34.793, 1.1465)
  line L2595 (34.793, 1.1465) -> (34.8128, 1.1438)
  line L2596 (34.8128, 1.1438) -> (34.8329, 1.1408)
  line L2597 (34.8329, 1.1408) -> (34.8528, 1.1375)
  line L2598 (34.8528, 1.1375) -> (34.8726, 1.1339)
  line L2599 (34.8726, 1.1339) -> (34.8922, 1.1298)
  line L2600 (34.8922, 1.1298) -> (34.912, 1.1255)
  line L2601 (34.912, 1.1255) -> (34.9316, 1.1208)
  line L2602 (34.9316, 1.1208) -> (34.9512, 1.1157)
  line L2603 (34.9512, 1.1157) -> (34.9705, 1.1103)
  line L2604 (34.9705, 1.1103) -> (34.9898, 1.1046)
  line L2605 (34.9898, 1.1046) -> (35.0091, 1.0985)
  line L2606 (35.0091, 1.0985) -> (35.0282, 1.0921)
  line L2607 (35.0282, 1.0921) -> (35.0472, 1.0854)
  line L2608 (35.0472, 1.0854) -> (35.066, 1.0783)
  line L2609 (35.066, 1.0783) -> (35.0848, 1.071)
  line L2610 (35.0848, 1.071) -> (35.1036, 1.0632)
  line L2611 (35.1036, 1.0632) -> (35.1219, 1.0552)
  line L2612 (35.1219, 1.0552) -> (35.1404, 1.0468)
  line L2613 (35.1404, 1.0468) -> (35.1586, 1.0382)
  line L2614 (35.1586, 1.0382) -> (35.1766, 1.0292)
  line L2615 (35.1766, 1.0292) -> (35.1943, 1.0199)
  line L2616 (35.1943, 1.0199) -> (35.2121, 1.0102)
  line L2617 (35.2121, 1.0102) -> (35.2298, 1.0003)
  line L2618 (35.2298, 1.0003) -> (35.247, 0.9901)
  line L2619 (35.247, 0.9901) -> (35.2642, 0.9796)
  line L2620 (35.2642, 0.9796) -> (35.2811, 0.9687)
  line L2621 (35.2811, 0.9687) -> (35.2981, 0.9576)
  line L2622 (35.2981, 0.9576) -> (35.3147, 0.9462)
  line L2623 (35.3147, 0.9462) -> (35.3311, 0.9345)
  line L2624 (35.3311, 0.9345) -> (35.3473, 0.9225)
  line L2625 (35.3473, 0.9225) -> (35.3632, 0.9102)
  line L2626 (35.3632, 0.9102) -> (35.379, 0.8977)
  line L2627 (35.379, 0.8977) -> (35.3946, 0.8848)
  line L2628 (35.3946, 0.8848) -> (35.41, 0.8717)
  line L2629 (35.41, 0.8717) -> (35.4251, 0.8584)
  line L2630 (35.4251, 0.8584) -> (35.4399, 0.8448)
  line L2631 (35.4399, 0.8448) -> (35.4544, 0.8309)
  line L2632 (35.4544, 0.8309) -> (35.469, 0.8168)
  line L2633 (35.469, 0.8168) -> (35.483, 0.8024)
  line L2634 (35.483, 0.8024) -> (35.497, 0.7878)
  line L2635 (35.497, 0.7878) -> (35.5105, 0.7729)
  line L2636 (35.5105, 0.7729) -> (35.524, 0.7578)
  line L2637 (35.524, 0.7578) -> (35.537, 0.7425)
  line L2638 (35.537, 0.7425) -> (35.5497, 0.7269)
  line L2639 (35.5497, 0.7269) -> (35.5624, 0.7111)
  line L2640 (35.5624, 0.7111) -> (35.5746, 0.6951)
  line L2641 (35.5746, 0.6951) -> (35.5867, 0.6789)
  line L2642 (35.5867, 0.6789) -> (35.5984, 0.6625)
  line L2643 (35.5984, 0.6625) -> (35.6097, 0.6459)
  line L2644 (35.6097, 0.6459) -> (35.6209, 0.6291)
  line L2645 (35.6209, 0.6291) -> (35.6317, 0.6121)
  line L2646 (35.6317, 0.6121) -> (35.6423, 0.5949)
  line L2647 (35.6423, 0.5949) -> (35.6523, 0.5775)
  line L2648 (35.6523, 0.5775) -> (35.6624, 0.56)
  line L2649 (35.6624, 0.56) -> (35.6719, 0.5423)
  line L2650 (35.6719, 0.5423) -> (35.6814, 0.5244)
  line L2651 (35.6814, 0.5244) -> (35.6904, 0.5063)
  line L2652 (35.6904, 0.5063) -> (35.6989, 0.4882)
  line L2653 (35.6989, 0.4882) -> (35.7074, 0.4698)
  line L2654 (35.7074, 0.4698) -> (35.7153, 0.4513)
  line L2655 (35.7153, 0.4513) -> (35.723, 0.4327)
  line L2656 (35.723, 0.4327) -> (35.7304, 0.4139)
  line L2657 (35.7304, 0.4139) -> (35.7375, 0.3951)
  line L2658 (35.7375, 0.3951) -> (35.7444, 0.3761)
  line L2659 (35.7444, 0.3761) -> (35.7508, 0.3569)
  line L2660 (35.7508, 0.3569) -> (35.7568, 0.3377)
  line L2661 (35.7568, 0.3377) -> (35.7624, 0.3184)
  line L2662 (35.7624, 0.3184) -> (35.768, 0.299)
  line L2663 (35.768, 0.299) -> (35.773, 0.2794)
  line L2664 (35.773, 0.2794) -> (35.7775, 0.2598)
  line L2665 (35.7775, 0.2598) -> (35.782, 0.2402)
  line L2666 (35.782, 0.2402) -> (35.786, 0.2204)
  line L2667 (35.786, 0.2204) -> (35.7897, 0.2006)
  line L2668 (35.7897, 0.2006) -> (35.7931, 0.1807)
  line L2669 (35.7931, 0.1807) -> (35.796, 0.1608)
  line L2670 (35.796, 0.1608) -> (35.7987, 0.1408)
  line L2671 (35.7987, 0.1408) -> (35.8008, 0.1207)
  line L2672 (35.8008, 0.1207) -> (35.8029, 0.1007)
  line L2673 (35.8029, 0.1007) -> (35.8045, 0.0806)
  line L2674 (35.8045, 0.0806) -> (35.8055, 0.0604)
  line L2675 (35.8055, 0.0604) -> (35.8066, 0.0403)
  line L2676 (35.8066, 0.0403) -> (35.8071, 0.0202)
  line L2677 (35.8071, 0.0202) -> (35.8071, 0)
  line L2678 (35.8071, 0) -> (35.8071, -0.0202)
  line L2679 (35.8071, -0.0202) -> (35.8066, -0.0403)
  line L2680 (35.8066, -0.0403) -> (35.8055, -0.0604)
  line L2681 (35.8055, -0.0604) -> (35.8045, -0.0806)
  line L2682 (35.8045, -0.0806) -> (35.8029, -0.1007)
  line L2683 (35.8029, -0.1007) -> (35.8008, -0.1207)
  line L2684 (35.8008, -0.1207) -> (35.7987, -0.1408)
  line L2685 (35.7987, -0.1408) -> (35.796, -0.1608)
  line L2686 (35.796, -0.1608) -> (35.7931, -0.1807)
  line L2687 (35.7931, -0.1807) -> (35.7897, -0.2006)
  line L2688 (35.7897, -0.2006) -> (35.786, -0.2204)
  line L2689 (35.786, -0.2204) -> (35.782, -0.2402)
  line L2690 (35.782, -0.2402) -> (35.7775, -0.2598)
  line L2691 (35.7775, -0.2598) -> (35.773, -0.2794)
  line L2692 (35.773, -0.2794) -> (35.768, -0.299)
  line L2693 (35.768, -0.299) -> (35.7624, -0.3184)
  line L2694 (35.7624, -0.3184) -> (35.7568, -0.3377)
  line L2695 (35.7568, -0.3377) -> (35.7508, -0.3569)
  line L2696 (35.7508, -0.3569) -> (35.7444, -0.3761)
  line L2697 (35.7444, -0.3761) -> (35.7375, -0.3951)
  line L2698 (35.7375, -0.3951) -> (35.7304, -0.4139)
  line L2699 (35.7304, -0.4139) -> (35.723, -0.4327)
  line L2700 (35.723, -0.4327) -> (35.7153, -0.4513)
  line L2701 (35.7153, -0.4513) -> (35.7074, -0.4698)
  line L2702 (35.7074, -0.4698) -> (35.6989, -0.4882)
  line L2703 (35.6989, -0.4882) -> (35.6904, -0.5063)
  line L2704 (35.6904, -0.5063) -> (35.6814, -0.5244)
  line L2705 (35.6814, -0.5244) -> (35.6719, -0.5423)
  line L2706 (35.6719, -0.5423) -> (35.6624, -0.56)
  line L2707 (35.6624, -0.56) -> (35.6523, -0.5775)
  line L2708 (35.6523, -0.5775) -> (35.6423, -0.5949)
  line L2709 (35.6423, -0.5949) -> (35.6317, -0.6121)
  line L2710 (35.6317, -0.6121) -> (35.6209, -0.6291)
  line L2711 (35.6209, -0.6291) -> (35.6097, -0.6459)
  line L2712 (35.6097, -0.6459) -> (35.5984, -0.6625)
  line L2713 (35.5984, -0.6625) -> (35.5867, -0.6789)
  line L2714 (35.5867, -0.6789) -> (35.5746, -0.6951)
  line L2715 (35.5746, -0.6951) -> (35.5624, -0.7111)
  line L2716 (35.5624, -0.7111) -> (35.5497, -0.7269)
  line L2717 (35.5497, -0.7269) -> (35.537, -0.7425)
  line L2718 (35.537, -0.7425) -> (35.524, -0.7578)
  line L2719 (35.524, -0.7578) -> (35.5105, -0.7729)
  line L2720 (35.5105, -0.7729) -> (35.497, -0.7878)
  line L2721 (35.497, -0.7878) -> (35.483, -0.8024)
  line L2722 (35.483, -0.8024) -> (35.469, -0.8168)
  line L2723 (35.469, -0.8168) -> (35.4544, -0.8309)
  line L2724 (35.4544, -0.8309) -> (35.4399, -0.8448)
  line L2725 (35.4399, -0.8448) -> (35.4251, -0.8584)
  line L2726 (35.4251, -0.8584) -> (35.41, -0.8717)
  line L2727 (35.41, -0.8717) -> (35.3946, -0.8848)
  line L2728 (35.3946, -0.8848) -> (35.379, -0.8977)
  line L2729 (35.379, -0.8977) -> (35.3632, -0.9102)
  line L2730 (35.3632, -0.9102) -> (35.3473, -0.9225)
  line L2731 (35.3473, -0.9225) -> (35.3311, -0.9345)
  line L2732 (35.3311, -0.9345) -> (35.3147, -0.9462)
  line L2733 (35.3147, -0.9462) -> (35.2981, -0.9576)
  line L2734 (35.2981, -0.9576) -> (35.2811, -0.9687)
  line L2735 (35.2811, -0.9687) -> (35.2642, -0.9796)
  line L2736 (35.2642, -0.9796) -> (35.247, -0.9901)
  line L2737 (35.247, -0.9901) -> (35.2298, -1.0003)
  line L2738 (35.2298, -1.0003) -> (35.2121, -1.0102)
  line L2739 (35.2121, -1.0102) -> (35.1943, -1.0199)
  line L2740 (35.1943, -1.0199) -> (35.1766, -1.0292)
  line L2741 (35.1766, -1.0292) -> (35.1586, -1.0382)
  line L2742 (35.1586, -1.0382) -> (35.1404, -1.0468)
  line L2743 (35.1404, -1.0468) -> (35.1219, -1.0552)
  line L2744 (35.1219, -1.0552) -> (35.1036, -1.0632)
  line L2745 (35.1036, -1.0632) -> (35.0848, -1.071)
  line L2746 (35.0848, -1.071) -> (35.066, -1.0783)
  line L2747 (35.066, -1.0783) -> (35.0472, -1.0854)
  line L2748 (35.0472, -1.0854) -> (35.0282, -1.0921)
  line L2749 (35.0282, -1.0921) -> (35.0091, -1.0985)
  line L2750 (35.0091, -1.0985) -> (34.9898, -1.1046)
  line L2751 (34.9898, -1.1046) -> (34.9705, -1.1103)
  line L2752 (34.9705, -1.1103) -> (34.9512, -1.1157)
  line L2753 (34.9512, -1.1157) -> (34.9316, -1.1208)
  line L2754 (34.9316, -1.1208) -> (34.912, -1.1255)
  line L2755 (34.912, -1.1255) -> (34.8922, -1.1298)
  line L2756 (34.8922, -1.1298) -> (34.8726, -1.1339)
  line L2757 (34.8726, -1.1339) -> (34.8528, -1.1375)
  line L2758 (34.8528, -1.1375) -> (34.8329, -1.1408)
  line L2759 (34.8329, -1.1408) -> (34.8128, -1.1438)
  line L2760 (34.8128, -1.1438) -> (34.793, -1.1465)
  line L2761 (34.793, -1.1465) -> (34.7729, -1.1487)
  line L2762 (34.7729, -1.1487) -> (34.7528, -1.1507)
  line L2763 (34.7528, -1.1507) -> (34.7326, -1.1523)
  line L2764 (34.7326, -1.1523) -> (34.7125, -1.1535)
  line L2765 (34.7125, -1.1535) -> (34.6924, -1.1544)
  line L2766 (34.6924, -1.1544) -> (34.6723, -1.1549)
  line L2767 (34.6723, -1.1549) -> (34.6522, -1.1551)
  line L2768 (34.6522, -1.1551) -> (34.6321, -1.1549)
extrude "Extrude1" add sketch "Sketch1" along normal blind 3.175
